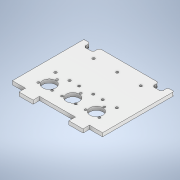
# Autodesk Inventor part: front_wall
Saved by Autodesk Inventor 2020 (Build 240168000, 168)
## iProperties
Created: 2019-06-12
Part Number: front_wall
Material: PPS Plastic
Document SubType Name: Modeling
Designer: Dammy
Density: 1.637 g/cm^3
Appearance: Smooth - White
Author: Dammy
Autodesk Inventor part; units mm, degrees
ref_plane "YZ Plane" through (0, 0, 0) normal (1, 0, 0) x (0, 1, 0)
ref_plane "XZ Plane" through (0, 0, 0) normal (0, 1, 0) x (-1, 0, 0)
ref_plane "XY Plane" through (0, 0, 0) normal (0, 0, 1) x (1, 0, 0)
sketch "Sketch1" plane through (0, 0, 0) normal (0, 1, 0) x (-1, 0, 0)
  line L0 (-41.5, -48.85) -> (-41.5, -45.85)
  line L1 (-44.5, -42.85) -> (-51.2, -42.85)
  line L2 (-54.2, -45.85) -> (-54.2, -48.85)
  line L3 (-57.2, -51.85) -> (-61.5, -51.85)
  arc A0 (-41.5, -48.85) -> (-38.5, -51.85) centre (-38.5, -48.85) ccw
  arc A1 (-41.5, -45.85) -> (-44.5, -42.85) centre (-44.5, -45.85) ccw
  arc A2 (-51.2, -42.85) -> (-54.2, -45.85) centre (-51.2, -45.85) ccw
  arc A3 (-57.2, -51.85) -> (-54.2, -48.85) centre (-57.2, -48.85) ccw
  line L4 (41.5, -48.85) -> (41.5, -45.85)
  line L5 (44.5, -42.85) -> (51.2, -42.85)
  line L6 (54.2, -45.85) -> (54.2, -48.85)
  line L7 (61.5, -51.85) -> (57.2, -51.85)
  line L8 (38.5, -51.85) -> (-38.5, -51.85)
  arc A4 (54.2, -48.85) -> (57.2, -51.85) centre (57.2, -48.85) ccw
  arc A5 (54.2, -45.85) -> (51.2, -42.85) centre (51.2, -45.85) ccw
  arc A6 (44.5, -42.85) -> (41.5, -45.85) centre (44.5, -45.85) ccw
  arc A7 (38.5, -51.85) -> (41.5, -48.85) centre (38.5, -48.85) ccw
  line L9 (44.75, 48.15) -> (25.05, 48.15)
  line L10 (25.05, 48.15) -> (25.05, 57.15)
  line L11 (25.05, 57.15) -> (44.75, 57.15)
  line L12 (44.75, 57.15) -> (44.75, 48.15)
  line L13 (-25.05, 48.15) -> (-44.75, 48.15)
  line L14 (-44.75, 48.15) -> (-44.75, 57.15)
  line L15 (-44.75, 57.15) -> (-25.05, 57.15)
  line L16 (-25.05, 57.15) -> (-25.05, 48.15)
  line L17 (44.75, 48.15) -> (63, 48.15)
  line L18 (25.05, 48.15) -> (-25.05, 48.15)
  line L19 (-44.75, 48.15) -> (-63, 48.15)
  line L20 (63, -50.35) -> (63, 48.15)
  line L21 (-63, -50.35) -> (-63, 48.15)
  arc A8 (61.5, -51.85) -> (63, -50.35) centre (61.5, -50.35) ccw
  arc A9 (-63, -50.35) -> (-61.5, -51.85) centre (-61.5, -50.35) ccw
  point P0 (0, 0)
  point P1 (-47.85, -48.15)
  point P2 (47.85, -48.85)
  point P3 (34.9, 57.15)
  point P4 (-34.9, 57.15)
  point P5 (-59.35, -51.85)
  point P6 (0, -51.85)
  point P7 (59.35, -51.85)
  point P8 (0, 48.15)
  point P9 (-47.85, -42.85)
  point P10 (47.85, -42.85)
  dimension "d3" = 12.7
  dimension "d5" = 3
  dimension "d7" = 12.7
  dimension "d9" = 3
  dimension "d10" = 9
  dimension "d11" = 19.7
  dimension "d13" = 9
  dimension "d14" = 19.7
  dimension "d16" = 1.5
  dimension "d17" = 126
  dimension "d20" = 18.25
  dimension "d21" = 18.25
  dimension "d22" = 57.15
  dimension "d23" = 9
  dimension "d24" = 9
  dimension "d27" = 91
  dimension "d28" = 91
  dimension "d53" = 83
  dimension "d54" = 3.7
  constraints: 44 end point, 20 point on circle, 19 tangent, 10 centre point, 10 parallel, 8 midpoint, 7 equal radius, 7 horizontal alignment, 4 horizontal, 4 vertical alignment, 3 perpendicular, 2 vertical, 1 collinear, 1 point on line
  measures "d3" distance between parallel lines of L2 L0
  measures "d5" radius of A0
  measures "d7" distance between parallel lines of L4 L6
  measures "d9" radius of A4
  measures "d10" distance between parallel lines of L9 L11
  measures "d11" distance of L9.start L9.end
  measures "d13" distance between parallel lines of L13 L15
  measures "d14" distance between parallel lines of L14 L16
  measures "d16" radius of A8
  measures "d17" distance between parallel lines of L21 L20
  measures "d20" distance between parallel lines of L20 L12
  measures "d21" distance between parallel lines of L21 L14
  measures "d22" distance from line of point (0, 0) L11
  measures "d23" distance between parallel lines of L8 L5
  measures "d24" distance between parallel lines of L8 L1
  measures "d27" distance between parallel lines of L5 L9
  measures "d28" distance between parallel lines of L13 L1
  measures "d53" distance between parallel lines of L0 L4
  measures "d54" distance from line of point (-47.85, -48.15) L7
extrude "base" add sketch "Sketch1" along normal blind 5
sketch "Sketch2" plane through (0, 5, 0) normal (0, 1, 0) x (1, 0, 0)
  circle A0 centre (0, -26.65) radius 9
  line L0 (-25.05, -48.15) -> (25.05, -48.15) projected
  line L1 (0, -26.65) -> (-33, -26.65) construction
  point P0 (0, 0)
  dimension "d31" = 18
  dimension "d32" = 21.5
  dimension "d52" = 33
  constraints: 2 end point, 1 centre point, 1 horizontal, 1 vertical alignment
  measures "d31" diameter of A0
  measures "d32" distance from line of L0 L1.start
  measures "d52" distance of L1.start L1.end
extrude "Poke Hole" cut sketch "Sketch2" against normal up to surface (5 mm away)
pattern_linear "Rectangular Pattern1" count 2 spacing 33 along (-1, 0, 0) count 2 spacing 33 along (1, 0, 0) of "Poke Hole"
sketch "Sketch3" plane through (0, 5, 0) normal (0, 1, 0) x (1, 0, 0)
  circle A0 centre (-33, -15.55) radius 1.5
  circle A1 centre (-33, -26.65) radius 9 projected
  circle A2 centre (-42.6129, -32.2) radius 1.5
  circle A3 centre (-23.3871, -32.2) radius 1.5
  point P0 (0, 0)
  dimension "d41" = 3
  dimension "d42" = 11.1
  dimension "d45" = 360
  constraints: 3 centre point, 1 coincident, 1 vertical alignment, 7 other
  measures "d41" diameter of A0
  measures "d42" distance of A1.centre A0.centre
extrude "Mount Holes" cut sketch "Sketch3" against normal up to surface (5 mm away) contours A0 | A2 | A3
pattern_linear "Rectangular Pattern2" count 3 spacing 33 along (1, 0, 0) of "Mount Holes"
sketch "Sketch4" plane through (0, 5, 0) normal (0, 1, 0) x (1, 0, 0)
  circle A0 centre (-42.875, -8.05) radius 1.65
  circle A1 centre (-23.125, -8.05) radius 1.65
  line L0 (-42.875, -8.05) -> (-23.125, -8.05) construction
  circle A2 centre (-33, -15.55) radius 1.5 construction
  circle A3 centre (-33, 35.3405) radius 1.65
  point P0 (0, 0)
  point P1 (-33, -8.05)
  dimension "d55" = 3.3
  dimension "d56" = 3.3
  dimension "d57" = 19.75
  dimension "d58" = 3.3
  dimension "d59" = 44.5
  dimension "d61" = 7.5
  constraints: 3 centre point, 2 end point, 2 vertical alignment, 1 coincident, 1 horizontal, 1 midpoint
  measures "d55" diameter of A0
  measures "d56" diameter of A1
  measures "d57" distance of L0.end L0.start
  measures "d58" diameter of A3
  measures "d59" distance of A3.centre L0.end
  measures "d61" distance of point (-33, -8.05) A2.centre
extrude "PCB mount holes" cut sketch "Sketch4" against normal up to surface (5 mm away)
pattern_linear "Rectangular Pattern3" count 3 spacing 33 along (1, 0, 0) of "PCB mount holes"
equation "\"d7\" = d3"
equation "\"d9\" = d5"
equation "\"d10\" = d23"
equation "\"d13\" = d23"
equation "\"d14\" = d11"
equation "\"d21\" = d20"
equation "\"d24\" = d23"
equation "\"d37\" = d52"
equation "\"d40\" = d52"
equation "\"d51\" = d52"
equation "\"d56\" = d55"
equation "\"d58\" = d55"
equation "\"d66\" = d52"
body "Solid1"
